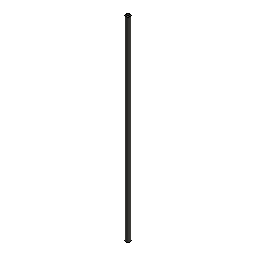
Tija (Autodesk Fusion 360 design; units mm, degrees)
part number: 2026-05-28-21-26-40-554
Autodesk Fusion 360 part; units mm, degrees
sketch "Sketch1" plane through (0, 0, 0) normal (0, 0, 1) x (1, 0, 0)
  circle A0 centre (8.6658, 10.0855) radius 1.15
  dimension "d1" = 2.3
  measures "d1" diameter of A0
extrude "Extrude1" add sketch "Sketch1" along normal blind 120
extrude "Extrude2" cut 1 faces at (8.9089, 10.1799, 120) along direction (0, 0, -1) blind 20
chamfer "Chamfer1" distance 0.5 angle 45 2 faces at (8.9089, 10.1799, 100) (9.7701, 9.7644, 33.3333)
